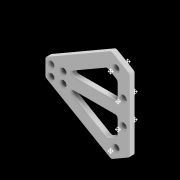
# Autodesk Inventor part: ShoulderBracket
Saved by Autodesk Inventor 2020 (Build 240168000, 168)
## iProperties
Created: 2020-04-01
Part Number: ShoulderBracket
Material: Generic
Document SubType Name: Modeling
Designer: valer
Density: 1 g/cm^3
Appearance: Default
Author: valer
Autodesk Inventor part; units mm, degrees
ref_plane "YZ Plane" through (0, 0, 0) normal (1, 0, 0) x (0, 1, 0)
ref_plane "XZ Plane" through (0, 0, 0) normal (0, 1, 0) x (-1, 0, 0)
ref_plane "XY Plane" through (0, 0, 0) normal (0, 0, 1) x (1, 0, 0)
sketch "Base" plane through (0, 0, 0) normal (0, 0, 1) x (1, 0, 0)
  line L0 (-88.9, 9.2829) -> (-88.9, -9.2829)
  line L1 (0, 38.1) -> (-19.4937, 49.3547)
  line L2 (-19.4937, -49.3547) -> (0, -38.1)
  line L3 (-88.9, 9.2829) -> (-19.4937, 49.3547)
  line L4 (-88.9, -9.2829) -> (-19.4937, -49.3547)
  line L5 (0, 38.1) -> (0, -38.1)
  line L6 (-68.58, -6.35) -> (-12.7, -6.35)
  line L7 (-12.7, -6.35) -> (-12.7, -38.6123)
  line L8 (-12.7, -38.6123) -> (-68.58, -6.35)
  line L9 (-88.9, 0) -> (0, 0) construction
  line L10 (-68.58, 6.35) -> (-12.7, 6.35)
  line L11 (-12.7, 6.35) -> (-12.7, 38.6123)
  line L12 (-12.7, 38.6123) -> (-68.58, 6.35)
  dimension "d0" = 120
  dimension "d1" = 60
  dimension "d2" = 120
  dimension "d3" = 60
  dimension "d4" = 12.7
  dimension "d5" = 12.7
  dimension "d6" = 20.32
  dimension "d7" = 12.7
  dimension "d9" = 120
  dimension "d10" = 120
  dimension "d11" = 76.2
  dimension "d12" = 88.9
  constraints: 26 end point, 3 parallel, 3 symmetric about line, 2 midpoint, 2 perpendicular, 1 coincident, 1 vertical
  measures "d0" angle of L5 L2
  measures "d1" angle of L5 L4
  measures "d2" angle of L1 L5
  measures "d3" angle of L5 L3
  measures "d4" distance between parallel lines of L5 L7
  measures "d5" distance between parallel lines of L4 L8
  measures "d6" distance from line of L0 L6.start
  measures "d7" distance between parallel lines of L6 L10
  measures "d9" angle of L1 L3
  measures "d10" angle of L2 L4
  measures "d11" distance of L1.start L2.end
  measures "d12" distance between parallel lines of L0 L5
extrude "BaseFeature" add sketch "Base" along normal blind 5.08
fillet "Fillet1" radius 2.54 6 edges at (-19.4937, 49.3547, 2.54) (0, 38.1, 2.54) (-19.4937, -49.3547, 2.54) (0, -38.1, 2.54) (-88.9, 9.2829, 2.54) (-88.9, -9.2829, 2.54)
fillet "Fillet2" radius 2.54 2 edges at (-68.58, 6.35, 2.54) (-68.58, -6.35, 2.54)
fillet "Fillet3" radius 2.54 2 edges at (-12.7, 6.35, 2.54) (-12.7, -6.35, 2.54)
chamfer "Chamfer1" distance 12.7 angle 45 2 edges at (-12.7, 38.6123, 2.54) (-12.7, -38.6123, 2.54)
fillet "Fillet4" radius 3.175 4 edges at (-23.6985, 32.2623, 2.54) (-12.7, 25.9123, 2.54) (-23.6985, -32.2623, 2.54) (-12.7, -25.9123, 2.54)
sketch "Sketch2" plane through (0, 0, 5.08) normal (0, 0, 1) x (1, 0, 0)
  circle A0 centre (-13.9731, -36.4073) radius 3.175
  circle A1 centre (-6.35, -12.7) radius 3.175
  line L0 (-12.7, -6.35) -> (-12.7, -38.6123) construction
  line L1 (0, -36.6335) -> (0, 36.6335) construction
  line L2 (-18.2237, -48.6215) -> (-1.27, -38.8332) construction
  line L3 (-88.9, 7.8165) -> (-88.9, -7.8165) construction
  line L4 (-88.9, 0) -> (0, 0) construction
  line L5 (0, -36.6335) -> (0, 36.6335) construction
  line L6 (-13.9731, -36.4073) -> (-9.7468, -43.7273) construction
  line L7 (-18.2237, -48.6215) -> (-1.27, -38.8332) construction
  line L8 (-20.7637, 48.6215) -> (-87.63, 10.0162) construction
  line L9 (-82.55, 12.9491) -> (-82.55, -12.9491) construction
  line L10 (-87.63, -10.0162) -> (-20.7637, -48.6215) construction
  arc A2 (-87.63, 10.0162) -> (-88.9, 7.8165) centre (-82.55, 5.6168) ccw construction
  circle A3 centre (-82.55, 5.6168) radius 3.175
  circle A4 centre (-82.55, -5.6168) radius 3.175
  circle A5 centre (-13.9731, 36.4073) radius 3.175
  circle A6 centre (-6.35, 12.7) radius 3.175
  circle A7 centre (-69.85, 5.6168) radius 3.175
  circle A8 centre (-69.85, -5.6168) radius 3.175
  line L11 (-82.55, 5.6168) -> (-69.85, 5.6168) construction
  line L12 (-69.85, 5.6168) -> (-69.85, -5.6168) construction
  line L13 (-69.85, -5.6168) -> (-82.55, -5.6168) construction
  line L14 (-1.27, 38.8332) -> (-18.2237, 48.6215) projected
  line L15 (-14.2875, 26.8289) -> (-22.111, 31.3458) projected
  dimension "d17" = 6.35
  dimension "d18" = 6.35
  dimension "d19" = 6.35
  dimension "d20" = 8.4524
  dimension "d23" = 6.35
  dimension "d27" = 11.2335
  dimension "d28" = 25.4
  dimension "d29" = 6.35
  dimension "d30" = 12.7
  dimension "d35" = 8.4524
  dimension "d36" = 8.4524
  constraints: 12 end point, 9 centre point, 4 equal radius, 4 perpendicular, 3 symmetric about line, 2 midpoint, 2 point on circle, 2 point on line, 2 vertical, 1 coincident, 3 other
  measures "d17" diameter of A1
  measures "d18" distance from line of L1 A1.centre
  measures "d19" distance from line of L0 A1.centre
  measures "d20" distance from line of L2 L6.start
  measures "d23" distance between parallel lines of L3 L9
  measures "d27" distance of L13.end A3.centre
  measures "d28" distance of A1.centre A6.centre
  measures "d29" distance from line of L3 L11.start
  measures "d30" distance between parallel lines of L9 L12
  measures "d35" distance from line of L14 A5.centre
  measures "d36" distance from line of L15 A5.centre
extrude "Extrusion2" cut sketch "Sketch2" against normal through all
ref_plane "Work Plane1" through (0, 0, 11.43) normal (0, 0, 1) x (1, 0, 0)
sketch "Sketch3" plane through (0, 0, 11.43) normal (0, 0, 1) x (1, 0, 0)
  circle A0 centre (-6.35, -12.7) radius 3.175 projected
  circle A1 centre (-6.35, 12.7) radius 3.175 projected
  circle A2 centre (-13.9731, 36.4073) radius 3.175 projected
  circle A3 centre (-13.9731, -36.4073) radius 3.175 projected
  circle A4 centre (-13.9731, -36.4073) radius 3.175 projected
  point P0 (0, 0)
  constraints: 4 coincident
ref_plane "Work Plane2" through (0, 0, -6.35) normal (0, 0, -1) x (-1, 0, 0)
sketch "Sketch4" plane through (0, 0, -6.35) normal (0, 0, -1) x (-1, 0, 0)
  circle A0 centre (13.9731, 36.4073) radius 3.175 projected
  circle A1 centre (6.35, 12.7) radius 3.175 projected
  circle A2 centre (6.35, -12.7) radius 3.175 projected
  circle A3 centre (13.9731, -36.4073) radius 3.175 projected
  point P0 (0, 0)
equation "\"d19\" = d18"
equation "\"d36\" = d35"
body "Solid1"
